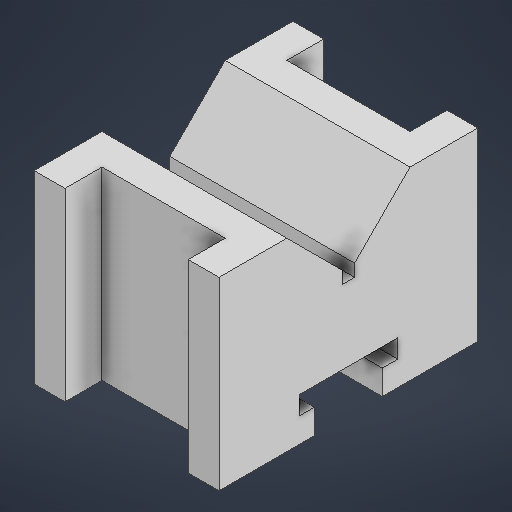
# Autodesk Inventor part: peca2
Saved by Autodesk Inventor 2026 (Build 300175050, 175E)
## iProperties
Created: 2026-04-30
Part Number: peca2
Material: Generic
Document SubType Name: Modeling
Designer: Administrator
Density: 1 g/cm^3
Appearance: Default
Author: Administrator
Autodesk Inventor part; units mm, degrees
ref_plane "YZ Plane" through (0, 0, 0) normal (1, 0, 0) x (0, 1, 0)
ref_plane "XZ Plane" through (0, 0, 0) normal (0, 1, 0) x (-1, 0, 0)
ref_plane "XY Plane" through (0, 0, 0) normal (0, 0, 1) x (1, 0, 0)
sketch "Sketch1" plane through (0, 0, 0) normal (1, 0, 0) x (0, 1, 0)
  line L0 (0, 0) -> (30, 0)
  line L1 (30, 0) -> (30, -11)
  line L2 (30, -11) -> (21, -20)
  line L3 (21, -20) -> (19, -20)
  line L4 (19, -20) -> (19, -22)
  line L5 (19, -22) -> (21, -22)
  line L6 (21, -22) -> (30, -31)
  line L7 (30, -31) -> (30, -42)
  line L8 (30, -42) -> (0, -42)
  line L9 (0, 0) -> (0, -42)
  dimension "d5" = 42
  dimension "d6" = 30
  dimension "d7" = 2
  dimension "d8" = 11
  dimension "d9" = 2
  dimension "d10" = 2
  dimension "d17" = 20
  dimension "d18" = 11
  constraints: 20 end point, 4 perpendicular, 2 horizontal, 2 point on line, 1 parallel, 1 vertical
  measures "d5" distance of L7.end L0.end
  measures "d6" distance of L7.end L8.end
  measures "d7" distance of L4.end L3.end
  measures "d8" horizontal distance of L7.end L4.end
  measures "d9" distance of L4.end L5.end
  measures "d10" distance of L2.end L3.end
  measures "d17" distance of L6.end L1.end
  measures "d18" distance of L0.end L1.end
extrude "Extrusion1" add sketch "Sketch1" against normal blind 30
sketch "Sketch2" plane through (0, 30, 0) normal (0, 1, 0) x (1, 0, 0)
  line L0 (0, 0) -> (-30, 0) projected
  line L1 (-25, 0) -> (-25, 6)
  line L2 (-25, 6) -> (-5, 6)
  line L3 (-5, 6) -> (-5, 0)
  line L4 (-30, 0) -> (-30, 11) projected
  line L5 (0, 11) -> (0, 0) projected
  line L6 (-25, 0) -> (-5, 0)
  line L7 (0, 42) -> (-30, 42) projected
  line L8 (-5, 42) -> (-5, 36)
  line L9 (-5, 36) -> (-25, 36)
  line L10 (-25, 36) -> (-25, 42)
  line L11 (-30, 31) -> (-30, 42) projected
  line L12 (0, 42) -> (0, 31) projected
  dimension "d13" = 5
  dimension "d14" = 5
  dimension "d21" = 30
  dimension "d22" = 6
  dimension "d23" = 5
  dimension "d24" = 5
  constraints: 14 end point, 4 perpendicular, 4 point on line, 2 vertical, 1 collinear
  measures "d13" distance between parallel lines of L4 L1
  measures "d14" distance between parallel lines of L5 L3
  measures "d21" distance between parallel lines of L2 L9
  measures "d22" distance between parallel lines of L0 L2
  measures "d23" distance between parallel lines of L11 L10
  measures "d24" distance between parallel lines of L12 L8
extrude "Extrusion2" cut sketch "Sketch2" against normal blind 30 contours L0 L1 L2 L3
extrude "Extrusion3" cut sketch "Sketch2" against normal blind 30 contours L8 L9 L10 L7
sketch "Sketch4" plane through (0, 0, 0) normal (1, 0, 0) x (0, 0, -1)
  line L0 (42, 0) -> (0, 0) projected
  line L1 (15.5, 0) -> (15.5, 4)
  line L2 (15.5, 4) -> (13, 4)
  line L3 (13, 4) -> (13, 7)
  line L4 (13, 7) -> (29, 7)
  line L5 (29, 7) -> (29, 4)
  line L6 (29, 4) -> (26.5, 4)
  line L7 (26.5, 4) -> (26.5, 0)
  line L8 (0, 30) -> (0, 0) projected
  line L9 (42, 0) -> (42, 30) projected
  line L10 (15.5, 0) -> (26.5, 0)
  dimension "d27" = 15.5
  dimension "d28" = 15.5
  dimension "d29" = 2.5
  dimension "d30" = 2.5
  dimension "d31" = 3
  dimension "d32" = 4
  constraints: 16 end point, 5 perpendicular, 4 point on line, 1 collinear, 1 vertical
  measures "d27" distance between parallel lines of L8 L1
  measures "d28" distance between parallel lines of L9 L7
  measures "d29" distance of L1.end L2.end
  measures "d30" distance of L5.end L6.end
  measures "d31" distance of L4.end L5.end
  measures "d32" distance of L6.end L7.end
extrude "Extrusion4" cut sketch "Sketch4" against normal blind 30
body "Solid1"
